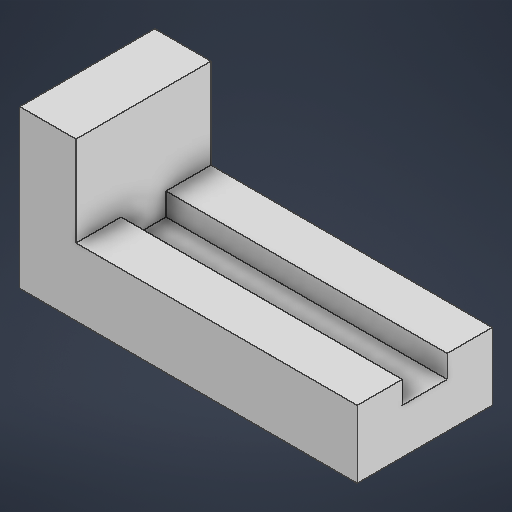
# Autodesk Inventor part: sabit_govde
Saved by Autodesk Inventor 2025.4 (Build 294407000, 407)
## iProperties
Created: 2026-06-17
Part Number: sabit_govde
Material: Generic
Document SubType Name: Modeling
Designer: yigithan
Density: 1 g/cm^3
Appearance: Default
Author: yigithan
Autodesk Inventor part; units mm, degrees
ref_plane "YZ Plane" through (0, 0, 0) normal (1, 0, 0) x (0, 1, 0)
ref_plane "XZ Plane" through (0, 0, 0) normal (0, 1, 0) x (-1, 0, 0)
ref_plane "XY Plane" through (0, 0, 0) normal (0, 0, 1) x (1, 0, 0)
sketch "Sketch1" plane through (0, 0, 0) normal (0, 0, 1) x (1, 0, 0)
  line L0 (0, 0) -> (150, 0)
  line L1 (150, 0) -> (150, 30)
  line L2 (150, 30) -> (25, 30)
  line L3 (25, 30) -> (25, 70)
  line L4 (25, 70) -> (0, 70)
  line L5 (0, 70) -> (0, 0)
  dimension "d0" = 150
  dimension "d1" = 30
  dimension "d2" = 125
  dimension "d3" = 40
  constraints: 12 end point, 5 perpendicular, 1 horizontal
  measures "d0" distance of L0.start L0.end
  measures "d1" distance of L0.end L1.end
  measures "d2" distance of L1.end L2.end
  measures "d3" distance of L2.end L3.end
extrude "Extrusion1" add sketch "Sketch1" along normal blind 60
sketch "Sketch2" plane through (150, 0, 0) normal (1, 0, 0) x (0, 0, -1)
  line L0 (0, 30) -> (-60, 30) projected
  line L1 (-40, 30) -> (-20, 30)
  line L2 (-20, 30) -> (-20, 20)
  line L3 (-20, 20) -> (-40, 20)
  line L4 (-40, 20) -> (-40, 30)
  point P0 (0, 0)
  dimension "d6" = 20
  dimension "d7" = 10
  constraints: 8 end point, 3 perpendicular, 2 point on line
  measures "d6" distance of L1.start L1.end
  measures "d7" distance of L1.end L2.end
extrude "Extrusion2" cut sketch "Sketch2" against normal blind 125
body "Solid1"
